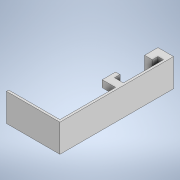
# Autodesk Inventor part: ESP_stand
Saved by Autodesk Inventor 2021 (Build 250183000, 183)
## iProperties
Created: 2021-03-18
Part Number: ESP_stand
Material: Generisch
Document SubType Name: Modeling
Designer: Tilman
Density: 1 g/cm^3
Appearance: Vorgabe
Author: Tilman
Autodesk Inventor part; units mm, degrees
ref_plane "YZ Plane" through (0, 0, 0) normal (1, 0, 0) x (0, 1, 0)
ref_plane "XZ Plane" through (0, 0, 0) normal (0, 1, 0) x (-1, 0, 0)
ref_plane "XY Plane" through (0, 0, 0) normal (0, 0, 1) x (1, 0, 0)
sketch "Skizze1" plane through (0, 0, 0) normal (0, 1, 0) x (-1, 0, 0)
  line L0 (0, 0) -> (-48, 0)
  line L1 (-48, 0) -> (-48, -102)
  line L2 (-48, -102) -> (-34, -102)
  line L3 (-34, -102) -> (-34, -52)
  line L4 (-34, -52) -> (-46, -52)
  line L5 (-46, -52) -> (-46, -2)
  line L6 (-46, -2) -> (0, -2)
  line L7 (0, -2) -> (0, 0)
  dimension "d0" = 2
  dimension "d1" = 46
  dimension "d2" = 48
  dimension "d3" = 50
  dimension "d4" = 50
  dimension "d5" = 12
  constraints: 16 end point, 6 perpendicular, 2 horizontal
  measures "d0" distance of L6.end L0.start
  measures "d1" distance of L5.end L6.end
  measures "d2" distance of L0.start L0.end
  measures "d3" distance of L4.end L5.end
  measures "d4" distance of L2.end L3.end
  measures "d5" distance of L3.end L4.end
extrude "Extrusion1" add sketch "Skizze1" along normal blind 25
sketch "Skizze2" plane through (0, 25, 0) normal (0, 1, 0) x (1, 0, 0)
  line L0 (48, 0) -> (48, 102) projected
  line L1 (48, 102) -> (34, 102) projected
  line L2 (34, 102) -> (34, 52) projected
  line L3 (34, 52) -> (46, 52) projected
  line L4 (46, 52) -> (46, 2) projected
  line L5 (46, 2) -> (0, 2) projected
  line L6 (0, 2) -> (0, 0) projected
  line L7 (0, 0) -> (48, 0) projected
  line L8 (46, 59) -> (46, 95)
  line L9 (46, 95) -> (41, 95)
  line L10 (41, 95) -> (41, 90)
  line L11 (41, 90) -> (34, 90)
  line L12 (34, 64) -> (38, 64)
  line L13 (38, 64) -> (38, 59)
  line L14 (38, 59) -> (46, 59)
  point P0 (34, 77)
  point P1 (46, 77)
  point P2 (39, 59)
  dimension "d18" = 5
  dimension "d19" = 36
  dimension "d20" = 5
  dimension "d21" = 8
  dimension "d22" = 5
  constraints: 14 end point, 4 perpendicular, 2 midpoint, 2 point on line, 2 vertical, 1 horizontal, 1 horizontal alignment, 1 vertical alignment
  measures "d18" distance of L8.end L9.end
  measures "d19" distance of L8.start L8.end
  measures "d20" distance of L9.end L10.end
  measures "d21" distance of L13.end L8.start
  measures "d22" distance of L12.end L13.end
extrude "Extrusion2" cut sketch "Skizze2" against normal through all contours L11 L10 L9 L8 L14 L13 L12 L2
sketch "Skizze3" plane through (34, 0, -52) normal (0, 0, 1) x (1, 0, 0)
  line L0 (0, 0) -> (12, 0) projected
  line L1 (12, 0) -> (12, 25) projected
  line L2 (0, 25) -> (12, 25) projected
  line L3 (0, 0) -> (0, 25) projected
  line L4 (12, 0) -> (12, 25) projected
  line L5 (12, 6.25) -> (0, 6.25)
  line L6 (0, 0) -> (0, 25) projected
  line L7 (0, 18.75) -> (12, 18.75)
  line L8 (6, 6.25) -> (6, 18.75) construction
  point P0 (-34, 0)
  point P1 (6, 12.5)
  point P2 (0, 12.5)
  dimension "d15" = 12.5
  constraints: 6 end point, 4 midpoint, 4 point on line, 2 horizontal, 1 horizontal alignment
  measures "d15" distance between parallel lines of L7 L5
extrude "Extrusion3" cut sketch "Skizze3" against normal up to surface (12 mm away) contours L3 L7 L1 L5
